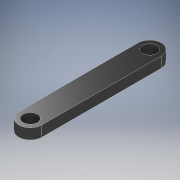
# Autodesk Inventor part: tuas
Saved by Autodesk Inventor 2021 (Build 250183000, 183)
## iProperties
Created: 2021-03-13
Part Number: tuas
Material: Generic
Document SubType Name: Modeling
Designer: Luthfi
Density: 1 g/cm^3
Appearance: Glossy - Black
Author: Luthfi
Autodesk Inventor part; units mm, degrees
ref_plane "YZ Plane" through (0, 0, 0) normal (1, 0, 0) x (0, 1, 0)
ref_plane "XZ Plane" through (0, 0, 0) normal (0, 1, 0) x (-1, 0, 0)
ref_plane "XY Plane" through (0, 0, 0) normal (0, 0, 1) x (1, 0, 0)
sketch "Sketch1" plane through (0, 0, 0) normal (0, 1, 0) x (-1, 0, 0)
  line L0 (0, 0) -> (0, -33.75) construction
  line L1 (-3.25, 0) -> (-3.25, -33.75)
  line L2 (3.25, -33.75) -> (3.25, 0)
  arc A0 (3.25, 0) -> (-3.25, 0) centre (0, 0) ccw
  arc A1 (-3.25, -33.75) -> (3.25, -33.75) centre (0, -33.75) ccw
  circle A2 centre (0, 0) radius 2
  circle A3 centre (0, -33.75) radius 2
  point P0 (0, -16.875)
  dimension "d0" = 33.75
  dimension "d1" = 6.5
  dimension "d2" = 4
  dimension "d3" = 4
  constraints: 8 end point, 4 centre point, 4 point on circle, 4 tangent, 2 coincident, 1 midpoint, 1 parallel, 1 vertical
  measures "d0" distance of L0.start L0.end
  measures "d1" diameter of A1
  measures "d2" diameter of A2
  measures "d3" diameter of A3
extrude "Extrusion1" add sketch "Sketch1" along normal blind 3
body "Solid1"
